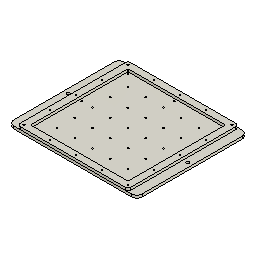
jig (Autodesk Fusion 360 design; units mm, degrees)
Autodesk Fusion 360 part; units mm, degrees
sketch "Sketch1" plane through (0, 0, 0) normal (0, 0, 1) x (1, 0, 0) in component "base"
  line L0 (62.5, 62.5) -> (-62.5, 62.5)
  line L1 (-62.5, 62.5) -> (-62.5, -62.5)
  line L2 (-62.5, -62.5) -> (62.5, -62.5)
  line L3 (62.5, -62.5) -> (62.5, 62.5)
  line L4 (62.5, 62.5) -> (-62.5, -62.5) construction
  line L5 (-62.5, 62.5) -> (62.5, -62.5) construction
  dimension "d3" = 125
  dimension "d4" = 125
  constraint horizontal L0
  constraint perpendicular L0 L1
  constraint parallel L0 L2
  constraint parallel L1 L3
  constraint coincident L4 origin
  constraint coincident L5 origin
  measures "d3" distance of L0.start L0.end
  measures "d4" distance of L0.start L2.end
extrude "Extrude1" add sketch "Sketch1" along normal blind 3 makes body 1 in component "base"
sketch "Sketch1 (2)" plane through (0, 0, 3) normal (0, 0, 1) x (-1, 0, 0) in component "stencilFrame"
  line L0 (-62.5, 62.5) -> (-62.5, -62.5)
  line L1 (-62.5, -62.5) -> (62.5, -62.5)
  line L2 (62.5, -62.5) -> (62.5, 62.5)
  line L3 (62.5, 62.5) -> (-62.5, 62.5)
  line L4 (-55, -55) -> (55, -55)
  line L5 (55, -55) -> (55, 55)
  line L6 (55, 55) -> (-55, 55)
  line L7 (-55, 55) -> (-55, -55)
  line L8 (-55, -55) -> (55, 55) construction
  line L9 (55, -55) -> (-55, 55) construction
  dimension "d7" = 110
  dimension "d8" = 110
  constraint horizontal L4
  constraint perpendicular L4 L5
  constraint parallel L4 L6
  constraint parallel L5 L7
  constraint coincident L8 origin
  constraint coincident L9 origin
  measures "d7" distance of L4.start L4.end
  measures "d8" distance of L4.start L6.end
extrude "Extrude1'" add sketch "Sketch1 (2)" along normal blind 3 separate body makes body 2 in component "stencilFrame"
sketch "Sketch2" plane through (0, 0, 3) normal (0, 0, 1) x (-1, 0, 0) in component "base"
  line L0 (-62.5, 62.5) -> (-62.5, -62.5)
  line L1 (-62.5, -62.5) -> (62.5, -62.5)
  line L2 (62.5, -62.5) -> (62.5, 62.5)
  line L3 (62.5, 62.5) -> (-62.5, 62.5)
hole "Hole1" at (0, 0, 3) direction (0, 0, -1) diameter 1.623 depth 40 tip angle 118 bodies 1 in component "base"
thread "Thread1" "ISO Metric profile 2.0 M2x0.4 6H" in component "base"
pattern_linear "R-Pattern1" count 5 spacing 20 along (1, 0, 0) both ways count 5 spacing 20 along (0, 1, 0) both ways of "Hole1" in component "base"
sketch "Sketch4" plane through (0, 0, 3) normal (0, 0, 1) x (-1, 0, 0) in component "base"
  circle A0 centre (-20, -20) radius 0.8115
  circle A1 centre (0, -20) radius 0.8115
  circle A2 centre (20, -20) radius 0.8115
  circle A3 centre (-20, 0) radius 0.8115
  circle A4 centre (20, 0) radius 0.8115
  circle A5 centre (-20, 20) radius 0.8115
  circle A6 centre (0, 20) radius 0.8115
  circle A7 centre (20, 20) radius 0.8115
  circle A8 centre (0, 0) radius 0.8115
  line L0 (-62.5, 62.5) -> (-62.5, -62.5)
  line L1 (-62.5, -62.5) -> (62.5, -62.5)
  line L2 (62.5, -62.5) -> (62.5, 62.5)
  line L3 (62.5, 62.5) -> (-62.5, 62.5)
  line L4 (-52.5, -52.5) -> (52.5, -52.5) construction
  line L5 (52.5, -52.5) -> (52.5, 52.5) construction
  line L6 (52.5, 52.5) -> (-52.5, 52.5) construction
  line L7 (-52.5, 52.5) -> (-52.5, -52.5) construction
  line L8 (-52.5, -52.5) -> (52.5, 52.5) construction
  line L9 (52.5, -52.5) -> (-52.5, 52.5) construction
  line L10 (55, -55) -> (-55, -55) construction
  line L11 (-55, -55) -> (-55, 55) construction
  circle A9 centre (-40, -20) radius 0.8115
  circle A10 centre (40, -20) radius 0.8115
  circle A11 centre (-40, 0) radius 0.8115
  circle A12 centre (40, 0) radius 0.8115
  circle A13 centre (-40, 20) radius 0.8115
  circle A14 centre (40, 20) radius 0.8115
  circle A15 centre (-40, -40) radius 0.8115
  circle A16 centre (-20, -40) radius 0.8115
  circle A17 centre (0, -40) radius 0.8115
  circle A18 centre (20, -40) radius 0.8115
  circle A19 centre (40, -40) radius 0.8115
  circle A20 centre (-40, 40) radius 0.8115
  circle A21 centre (-20, 40) radius 0.8115
  circle A22 centre (0, 40) radius 0.8115
  circle A23 centre (20, 40) radius 0.8115
  circle A24 centre (40, 40) radius 0.8115
  point P0 (0, -52.5)
  point P1 (-52.5, 0)
  point P2 (0, 52.5)
  point P3 (52.5, 0)
  dimension "d28" = 2.5
  dimension "d29" = 2.5
  constraint horizontal L4
  constraint perpendicular L4 L5
  constraint parallel L4 L6
  constraint parallel L5 L7
  constraint coincident L8 A8.centre
  constraint coincident L9 A8.centre
  constraint coincident A8.centre origin
  constraint midpoint L4 P0
  constraint midpoint L7 P1
  constraint midpoint L6 P2
  constraint midpoint L5 P3
  measures "d28" distance of L4 L10
  measures "d29" distance of L7 L11
hole "Hole3" at (-52.5, 52.5, 3) at (52.5, 52.5, 3) at (52.5, -52.5, 3) at (-52.5, -52.5, 3) at (0, 52.5, 3) at (52.5, 0, 3) at (0, -52.5, 3) at (-52.5, 0, 3) direction (0, 0, -1) diameter 1.623 depth 40 tip angle 118 bodies 1 in component "base"
thread "Thread3" "ISO Metric profile 2.0 M2x0.4 6H" in component "base"
sketch "Sketch2 (2)" plane through (0, 0, 6) normal (0, 0, 1) x (-1, 0, 0) in component "stencilFrame"
  line L0 (-55, -55) -> (-55, 55)
  line L1 (-55, 55) -> (55, 55)
  line L2 (55, 55) -> (55, -55)
  line L3 (55, -55) -> (-55, -55)
  line L4 (62.5, 62.5) -> (-62.5, 62.5)
  line L5 (-62.5, 62.5) -> (-62.5, -62.5)
  line L6 (-62.5, -62.5) -> (62.5, -62.5)
  line L7 (62.5, -62.5) -> (62.5, 62.5)
  line L8 (-58.75, -58.75) -> (58.75, -58.75)
  line L9 (58.75, -58.75) -> (58.75, 58.75)
  line L10 (58.75, 58.75) -> (-58.75, 58.75)
  line L11 (-58.75, 58.75) -> (-58.75, -58.75)
  line L12 (-58.75, -58.75) -> (58.75, 58.75) construction
  line L13 (58.75, -58.75) -> (-58.75, 58.75) construction
  line L14 (0, -62.5) -> (0, -55) construction
  line L15 (55, 0) -> (62.5, 0) construction
  line L16 (29.375, -58.75) -> (29.375, 58.75) construction
  line L17 (-29.375, -58.75) -> (-29.375, 58.75) construction
  line L18 (58.75, -29.375) -> (-58.75, -29.375) construction
  line L19 (58.75, 29.375) -> (-58.75, 29.375) construction
  point P0 (58.75, 0)
  point P1 (-58.75, 0)
  point P2 (0, -58.75)
  point P3 (0, 58.75)
  dimension "d33" = 29.375
  dimension "d34" = 29.375
  dimension "d35" = 29.375
  dimension "d36" = 29.375
  constraint horizontal L8
  constraint perpendicular L8 L9
  constraint parallel L8 L10
  constraint parallel L9 L11
  constraint coincident L12 origin
  constraint coincident L13 origin
  constraint midpoint L6 L14.start
  constraint midpoint L3 L14.end
  constraint midpoint L8 L14
  constraint midpoint L2 L15.start
  constraint midpoint L7 L15.end
  constraint midpoint L9 L15
  constraint coincident L8 L16.start
  constraint coincident L10 L16.end
  constraint perpendicular L10 L16
  constraint coincident L8 L17.start
  constraint coincident L10 L17.end
  constraint perpendicular L10 L17
  constraint coincident L9 L18.start
  constraint coincident L11 L18.end
  constraint perpendicular L11 L18
  constraint coincident L9 L19.start
  constraint coincident L11 L19.end
  constraint perpendicular L11 L19
  constraint midpoint L15 P0
  constraint midpoint L11 P1
  constraint midpoint L14 P2
  constraint midpoint L10 P3
  measures "d33" distance of L9 L16
  measures "d34" distance of L11 L17
  measures "d35" distance of L8 L18
  measures "d36" distance of L10 L19
hole "Hole1'" at (-29.375, 58.75, 6) at (0, 58.75, 6) at (29.375, 58.75, 6) at (58.75, 29.375, 6) at (58.75, 0, 6) at (58.75, -29.375, 6) at (29.375, -58.75, 6) at (0, -58.75, 6) at (-29.375, -58.75, 6) at (-58.75, -29.375, 6) at (-58.75, 0, 6) at (-58.75, 29.375, 6) direction (0, 0, -1) diameter 1.623 depth 40 tip angle 118 bodies 2 in component "stencilFrame"
thread "Thread1'" "ISO Metric profile 2.0 M2x0.4 6H" in component "stencilFrame"
hole "Hole4" at (-58.75, 58.75, 6) at (58.75, 58.75, 6) at (58.75, -58.75, 6) at (-58.75, -58.75, 6) direction (0, 0, -1) diameter 2 depth 40 tip angle 180 bodies 1 in component "base"
hole "Hole2" at (-58.75, 58.75, 6) at (58.75, 58.75, 6) at (58.75, -58.75, 6) at (-58.75, -58.75, 6) direction (0, 0, -1) diameter 2 depth 40 tip angle 180 bodies 2 in component "stencilFrame"
sketch "Sketch1 (3)" plane through (0, 0, 0) normal (0, 0, -1) x (1, 0, 0) in component "aligmentPin"
  circle A0 centre (58.75, 58.75) radius 1
  circle A1 centre (-58.75, -58.75) radius 1
  circle A2 centre (58.75, -58.75) radius 1
  circle A3 centre (-58.75, 58.75) radius 1
  circle A4 centre (0, 52.5) radius 0.8115
  circle A5 centre (0, -52.5) radius 0.8115
  circle A6 centre (52.5, 52.5) radius 0.8115
  circle A7 centre (-52.5, -52.5) radius 0.8115
  circle A8 centre (52.5, -52.5) radius 0.8115
  circle A9 centre (-52.5, 52.5) radius 0.8115
  circle A10 centre (52.5, 0) radius 0.8115
  circle A11 centre (-52.5, 0) radius 0.8115
  circle A12 centre (20, -20) radius 0.8115
  circle A13 centre (0, -20) radius 0.8115
  circle A14 centre (-20, -20) radius 0.8115
  circle A15 centre (20, 0) radius 0.8115
  circle A16 centre (-20, 0) radius 0.8115
  circle A17 centre (20, 20) radius 0.8115
  circle A18 centre (0, 20) radius 0.8115
  circle A19 centre (-20, 20) radius 0.8115
  circle A20 centre (0, 0) radius 0.8115
  line L0 (62.5, -62.5) -> (62.5, 62.5)
  line L1 (62.5, 62.5) -> (-62.5, 62.5)
  line L2 (-62.5, 62.5) -> (-62.5, -62.5)
  line L3 (-62.5, -62.5) -> (62.5, -62.5)
  circle A21 centre (40, -20) radius 0.8115
  circle A22 centre (-40, -20) radius 0.8115
  circle A23 centre (40, 0) radius 0.8115
  circle A24 centre (-40, 0) radius 0.8115
  circle A25 centre (40, 20) radius 0.8115
  circle A26 centre (-40, 20) radius 0.8115
  circle A27 centre (40, -40) radius 0.8115
  circle A28 centre (20, -40) radius 0.8115
  circle A29 centre (0, -40) radius 0.8115
  circle A30 centre (-20, -40) radius 0.8115
  circle A31 centre (-40, -40) radius 0.8115
  circle A32 centre (40, 40) radius 0.8115
  circle A33 centre (20, 40) radius 0.8115
  circle A34 centre (0, 40) radius 0.8115
  circle A35 centre (-20, 40) radius 0.8115
  circle A36 centre (-40, 40) radius 0.8115
extrude "Extrude1''" add sketch "Sketch1 (3)" against normal blind 6 separate body contours A0 makes body 3 in component "aligmentPin"
fillet "Fillet1" radius 0.25 1 edges at (57.8177, -58.3884, 0) on bodies 3 in component "aligmentPin"
chamfer "Chamfer1" distance 0.2 distance2 0.8 1 edges at (57.8177, -59.1116, 6) measured on face at (58.9578, -59.11, 6) on bodies 3 in component "aligmentPin"
fillet "Fillet1'" radius 1 4 edges at (55, -55, 4.5) (55, 55, 4.5) (-55, 55, 4.5) (-55, -55, 4.5) on bodies 2 in component "stencilFrame"
fillet "Fillet1'" radius 3 4 edges at (-62.5, 62.5, 4.5) (-62.5, -62.5, 4.5) (62.5, -62.5, 4.5) (62.5, 62.5, 4.5) on bodies 2 in component "stencilFrame"
move_face "OffsetFaces1" offset 10 2 faces at (-62.5, 20.8333, 1) (62.5, -20.8333, 1) on bodies 1 in component "base"
sketch "Sketch5" plane through (0, 0, 3) normal (0, 0, 1) x (-1, 0, 0) in component "base"
  circle A0 centre (-58.75, 58.75) radius 1
  circle A1 centre (58.75, -58.75) radius 1
  circle A2 centre (-58.75, -58.75) radius 1
  circle A3 centre (58.75, 58.75) radius 1
  circle A4 centre (0, 52.5) radius 0.8115
  circle A5 centre (0, -52.5) radius 0.8115
  circle A6 centre (-52.5, 52.5) radius 0.8115
  circle A7 centre (52.5, -52.5) radius 0.8115
  circle A8 centre (-52.5, -52.5) radius 0.8115
  circle A9 centre (52.5, 52.5) radius 0.8115
  circle A10 centre (-52.5, 0) radius 0.8115
  circle A11 centre (52.5, 0) radius 0.8115
  circle A12 centre (-20, -20) radius 0.8115
  circle A13 centre (0, -20) radius 0.8115
  circle A14 centre (20, -20) radius 0.8115
  circle A15 centre (-20, 0) radius 0.8115
  circle A16 centre (20, 0) radius 0.8115
  circle A17 centre (-20, 20) radius 0.8115
  circle A18 centre (0, 20) radius 0.8115
  circle A19 centre (20, 20) radius 0.8115
  circle A20 centre (0, 0) radius 0.8115
  line L0 (-72.5, 62.5) -> (-72.5, -62.5)
  line L1 (-72.5, -62.5) -> (72.5, -62.5)
  line L2 (72.5, -62.5) -> (72.5, 62.5)
  line L3 (72.5, 62.5) -> (-72.5, 62.5)
  line L4 (72.5, -62.5) -> (72.5, 62.5) construction
  line L5 (62.5, -59.5) -> (62.5, 59.5) construction
  line L6 (-62.5, 59.5) -> (-62.5, -59.5) construction
  line L7 (-72.5, 62.5) -> (-72.5, -62.5) construction
  line L8 (62.5, 0) -> (72.5, 0)
  line L9 (-62.5, 0) -> (-72.5, 0)
  circle A21 centre (-40, -20) radius 0.8115
  circle A22 centre (40, -20) radius 0.8115
  circle A23 centre (-40, 0) radius 0.8115
  circle A24 centre (40, 0) radius 0.8115
  circle A25 centre (-40, 20) radius 0.8115
  circle A26 centre (40, 20) radius 0.8115
  circle A27 centre (-40, -40) radius 0.8115
  circle A28 centre (-20, -40) radius 0.8115
  circle A29 centre (0, -40) radius 0.8115
  circle A30 centre (20, -40) radius 0.8115
  circle A31 centre (40, -40) radius 0.8115
  circle A32 centre (-40, 40) radius 0.8115
  circle A33 centre (-20, 40) radius 0.8115
  circle A34 centre (0, 40) radius 0.8115
  circle A35 centre (20, 40) radius 0.8115
  circle A36 centre (40, 40) radius 0.8115
  point P0 (67.5, 0)
  point P1 (-67.5, 0)
  constraint midpoint L5 L8.start
  constraint midpoint L4 L8.end
  constraint midpoint L6 L9.start
  constraint midpoint L0 L9.end
  constraint midpoint L8 P0
  constraint midpoint L9 P1
hole "Hole5" at (-67.5, 0, 3) at (67.5, 0, 3) direction (0, 0, -1) diameter 3.5 depth 40 tip angle 180 bodies 1 in component "base"
fillet "Fillet1''" radius 6 4 edges at (-72.5, -62.5, 1.5) (72.5, -62.5, 1.5) (72.5, 62.5, 1.5) (-72.5, 62.5, 1.5) on bodies 1 in component "base"
component "base" placed x (1, 0, 0) y (0, 1, 0) z (0, 0, 1) at (0, 0, 0)
component "stencilFrame" placed x (1, 0, 0) y (0, 1, 0) z (0, 0, 1) at (0, 0, 0)
component "aligmentPin" placed x (1, 0, 0) y (0, 1, 0) z (0, 0, 1) at (0, 0, 0)
component "aligmentPin" placed x (1, 0, 0) y (0, 1, 0) z (0, 0, 1) at (0, 117.5, 0)
component "aligmentPin" placed x (1, 0, 0) y (0, 1, 0) z (0, 0, 1) at (-117.5, 0, 0)
component "aligmentPin" placed x (1, 0, 0) y (0, 1, 0) z (0, 0, 1) at (-117.5, 117.5, 0)
equation "frameWidth = 100 mm"
equation "frameHeight = 100 mm"
equation "d3 = frameWidth + 25 mm"
equation "d4 = frameHeight + 25 mm"
equation "d7 = frameWidth + 10 mm"
equation "d8 = frameHeight + 10 mm"
equation "d14 = floor(( frameWidth + 10 mm ) / holeSpacing)"
equation "d15 = floor(( frameHeight + 10 mm ) / holeSpacing)"
equation "d16 = holeSpacing"
equation "d17 = holeSpacing"
equation "holeSpacing = 20 mm"
equation "d28 = ( 5 / 2 ) * 1 mm"
equation "d29 = d28"
equation "d33 = ( frameWidth + 17.5 mm ) / 4"
equation "d34 = d33"
equation "d35 = ( frameHeight + 17.5 mm ) / 4"
equation "d36 = d35"
